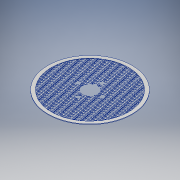
# Autodesk Inventor part: Ground_Antenna230mm_Reflector
Saved by Autodesk Inventor 2018 (Build 220112000, 112)
## iProperties
Created: 2018-09-26
Part Number: Ground_Antenna230mm_Reflector
Material: Aluminum 6061
Document SubType Name: Modeling
Designer: Bradley
Density: 2.7 g/cm^3
Appearance: Aluminum - Flat
Mass: 288.186 g
Surface Area: 2617.31 cm^2
Volume: 106.736 cm^3
Author: Bradley
Autodesk Inventor part; units mm, degrees
ref_plane "YZ Plane" through (0, 0, 0) normal (1, 0, 0) x (0, 1, 0)
ref_plane "XZ Plane" through (0, 0, 0) normal (0, 1, 0) x (-1, 0, 0)
ref_plane "XY Plane" through (0, 0, 0) normal (0, 0, 1) x (1, 0, 0)
sketch "Sketch1" plane through (0, 0, 0) normal (0, 0, 1) x (1, 0, 0)
  circle A0 centre (0, 0) radius 152.4
  circle A1 centre (0, 0) radius 139.7
  dimension "d0" = 304.8
  dimension "d1" = 279.4
  constraints: 2 centre point, 2 coincident
  measures "d0" diameter of A0
  measures "d1" diameter of A1
sketch "Sketch2" plane through (0, 0, 0) normal (0, 0, 1) x (1, 0, 0)
  line L0 (-152.4, 139.7) -> (152.4, 139.7)
  line L1 (152.4, 139.7) -> (152.4, 136.7)
  line L2 (152.4, 136.7) -> (-152.4, 136.7)
  line L3 (-152.4, 136.7) -> (-152.4, 139.7)
  circle A0 centre (0, 0) radius 139.7 projected
  line L4 (-152.4, 129.2) -> (152.4, 129.2)
  line L5 (152.4, 129.2) -> (152.4, 126.2)
  line L6 (152.4, 126.2) -> (-152.4, 126.2)
  line L7 (-152.4, 126.2) -> (-152.4, 129.2)
  line L8 (-152.4, 118.7) -> (152.4, 118.7)
  line L9 (152.4, 118.7) -> (152.4, 115.7)
  line L10 (152.4, 115.7) -> (-152.4, 115.7)
  line L11 (-152.4, 115.7) -> (-152.4, 118.7)
  line L12 (-152.4, 108.2) -> (152.4, 108.2)
  line L13 (152.4, 108.2) -> (152.4, 105.2)
  line L14 (152.4, 105.2) -> (-152.4, 105.2)
  line L15 (-152.4, 105.2) -> (-152.4, 108.2)
  line L16 (-152.4, 97.7) -> (152.4, 97.7)
  line L17 (152.4, 97.7) -> (152.4, 94.7)
  line L18 (152.4, 94.7) -> (-152.4, 94.7)
  line L19 (-152.4, 94.7) -> (-152.4, 97.7)
  line L20 (-152.4, 87.2) -> (152.4, 87.2)
  line L21 (152.4, 87.2) -> (152.4, 84.2)
  line L22 (152.4, 84.2) -> (-152.4, 84.2)
  line L23 (-152.4, 84.2) -> (-152.4, 87.2)
  line L24 (-152.4, 76.7) -> (152.4, 76.7)
  line L25 (152.4, 76.7) -> (152.4, 73.7)
  line L26 (152.4, 73.7) -> (-152.4, 73.7)
  line L27 (-152.4, 73.7) -> (-152.4, 76.7)
  line L28 (-152.4, 66.2) -> (152.4, 66.2)
  line L29 (152.4, 66.2) -> (152.4, 63.2)
  line L30 (152.4, 63.2) -> (-152.4, 63.2)
  line L31 (-152.4, 63.2) -> (-152.4, 66.2)
  line L32 (-152.4, 55.7) -> (152.4, 55.7)
  line L33 (152.4, 55.7) -> (152.4, 52.7)
  line L34 (152.4, 52.7) -> (-152.4, 52.7)
  line L35 (-152.4, 52.7) -> (-152.4, 55.7)
  line L36 (-152.4, 45.2) -> (152.4, 45.2)
  line L37 (152.4, 45.2) -> (152.4, 42.2)
  line L38 (152.4, 42.2) -> (-152.4, 42.2)
  line L39 (-152.4, 42.2) -> (-152.4, 45.2)
  point P0 (0, 139.7)
  point P1 (0, 129.2)
  point P2 (0, 118.7)
  point P3 (0, 108.2)
  point P4 (0, 97.7)
  point P5 (0, 87.2)
  point P6 (0, 76.7)
  point P7 (0, 66.2)
  point P8 (0, 55.7)
  point P9 (0, 45.2)
  dimension "d2" = 304.8
  dimension "d3" = 3
  dimension "d6" = 10.5
  constraints: 80 end point, 2 parallel, 1 collinear, 1 horizontal, 1 midpoint, 1 perpendicular, 1 tangent, 1 vertical, 1 vertical alignment, 80 other
  measures "d2" distance of L0.start L0.end
  measures "d3" distance of L0.end L1.end
  measures "d6" distance of L0.start L4.start
extrude "Extrusion1" add sketch "Sketch2" along normal mid plane 0.75 contours L0 A0 L2 L3 | L0 L1 L2 A0 | A0 L2 | L4 L5 L6 A0 | A0 L6 L4 | A0 L6 L7 L4 | L8 L9 L10 A0 | A0 L10 L8 | A0 L10 L11 L8 | L12 L13 L14 A0 | A0 L14 L12 | A0 L14 L15 L12 | L16 L17 L18 A0 | A0 L18 L16 | A0 L18 L19 L16 | L20 L21 L22 A0 | A0 L22 L20 | A0 L22 L23 L20 | L24 L25 L26 A0 | A0 L26 L24 | A0 L26 L27 L24 | L28 L29 L30 A0 | A0 L30 L28 | A0 L30 L31 L28 | L32 L33 L34 A0 | A0 L34 L32 | A0 L34 L35 L32 | L36 L37 L38 A0 | A0 L38 L36 | A0 L38 L39 L36
pattern_linear "Rectangular Pattern1" count 3 spacing 105 along (0, -1, 0) of "Extrusion1"
sketch "Sketch3" plane through (0, 0, 0) normal (0, 0, 1) x (1, 0, 0)
  line L0 (-201.8323, 44.7837) -> (62.1323, 197.1837)
  line L1 (62.1323, 197.1837) -> (63.6323, 194.5857)
  line L2 (63.6323, 194.5857) -> (-200.3323, 42.1857)
  line L3 (-200.3323, 42.1857) -> (-201.8323, 44.7837)
  line L4 (152.4, 139.7) -> (-152.4, 139.7) projected
  line L5 (152.4, 136.7) -> (152.4, 139.7) projected
  circle A0 centre (0, 0) radius 139.7 projected
  line L6 (0, 0) -> (-69.85, 120.9837)
  line L7 (-196.5823, 35.6905) -> (67.3823, 188.0905)
  line L8 (67.3823, 188.0905) -> (68.8823, 185.4924)
  line L9 (68.8823, 185.4924) -> (-195.0823, 33.0924)
  line L10 (-195.0823, 33.0924) -> (-196.5823, 35.6905)
  line L11 (-191.3323, 26.5972) -> (72.6323, 178.9972)
  line L12 (72.6323, 178.9972) -> (74.1323, 176.3991)
  line L13 (74.1323, 176.3991) -> (-189.8323, 23.9991)
  line L14 (-189.8323, 23.9991) -> (-191.3323, 26.5972)
  line L15 (-186.0823, 17.5039) -> (77.8823, 169.9039)
  line L16 (77.8823, 169.9039) -> (79.3823, 167.3059)
  line L17 (79.3823, 167.3059) -> (-184.5823, 14.9059)
  line L18 (-184.5823, 14.9059) -> (-186.0823, 17.5039)
  line L19 (-180.8323, 8.4107) -> (83.1323, 160.8107)
  line L20 (83.1323, 160.8107) -> (84.6323, 158.2126)
  line L21 (84.6323, 158.2126) -> (-179.3323, 5.8126)
  line L22 (-179.3323, 5.8126) -> (-180.8323, 8.4107)
  line L23 (-175.5823, -0.6826) -> (88.3823, 151.7174)
  line L24 (88.3823, 151.7174) -> (89.8823, 149.1193)
  line L25 (89.8823, 149.1193) -> (-174.0823, -3.2807)
  line L26 (-174.0823, -3.2807) -> (-175.5823, -0.6826)
  line L27 (-170.3323, -9.7759) -> (93.6323, 142.6241)
  line L28 (93.6323, 142.6241) -> (95.1323, 140.0261)
  line L29 (95.1323, 140.0261) -> (-168.8323, -12.3739)
  line L30 (-168.8323, -12.3739) -> (-170.3323, -9.7759)
  line L31 (-165.0823, -18.8691) -> (98.8823, 133.5309)
  line L32 (98.8823, 133.5309) -> (100.3823, 130.9328)
  line L33 (100.3823, 130.9328) -> (-163.5823, -21.4672)
  line L34 (-163.5823, -21.4672) -> (-165.0823, -18.8691)
  line L35 (-159.8323, -27.9624) -> (104.1323, 124.4376)
  line L36 (104.1323, 124.4376) -> (105.6323, 121.8395)
  line L37 (105.6323, 121.8395) -> (-158.3323, -30.5605)
  line L38 (-158.3323, -30.5605) -> (-159.8323, -27.9624)
  line L39 (-154.5823, -37.0557) -> (109.3823, 115.3443)
  line L40 (109.3823, 115.3443) -> (110.8823, 112.7463)
  line L41 (110.8823, 112.7463) -> (-153.0823, -39.6537)
  line L42 (-153.0823, -39.6537) -> (-154.5823, -37.0557)
  point P0 (-64.6, 111.8905)
  point P1 (-59.35, 102.7972)
  point P2 (-54.1, 93.7039)
  point P3 (-48.85, 84.6107)
  point P4 (-43.6, 75.5174)
  point P5 (-38.35, 66.4241)
  point P6 (-33.1, 57.3309)
  point P7 (-27.85, 48.2376)
  point P8 (-22.6, 39.1443)
  dimension "d23" = 30
  dimension "d26" = 10.5
  constraints: 82 end point, 2 equal length, 2 parallel, 1 collinear, 1 midpoint, 1 perpendicular, 84 other
  measures "d23" angle of L0 L4
  measures "d26" distance of L0.start L7.start
extrude "Extrusion4" add sketch "Sketch3" along normal mid plane 0.75 contours L0 A0 L2 L3 | L0 L4 L2 A0 | L6 L2 A0 | A0 L2 L6 | L0 L1 L2 L4 | L7 L4 L9 A0 | A0 L9 L6 L7 | L7 L6 L9 A0 | A0 L9 L10 L7 | L7 L8 L9 L4 | L11 L6 L13 A0 | A0 L13 L14 L11 | L11 A0 L13 L6 | L11 L12 L13 L4 | L4 L13 A0 L11 | L15 L6 L17 A0 | A0 L17 L18 L15 | L15 A0 L17 L6 | L15 L16 L17 L4 | L4 L17 A0 L15 | L19 L6 L21 A0 | A0 L21 L22 L19 | L19 A0 L21 L6 | L19 L20 L21 L4 | L4 L21 A0 L19 | L23 L6 L25 A0 | A0 L25 L26 L23 | L23 A0 L25 L6 | L23 L24 L25 L4 | L4 L25 A0 L23 | L27 L6 L29 A0 | A0 L29 L30 L27 | L27 A0 L29 L6 | L27 L28 L29 L4 | L4 L29 A0 L27 | L31 L6 L33 A0 | A0 L33 L34 L31 | L31 A0 L33 L6 | L31 L32 L33 A0 | L35 L6 L37 A0 | A0 L37 L38 L35 | L35 A0 L37 L6 | L35 L36 L37 A0 | L39 L6 L41 A0 | A0 L41 L42 L39 | L39 A0 L41 L6 | L39 L40 L41 A0
pattern_linear "Rectangular Pattern2" count 3 spacing 105 along (0.5, -0.866, 0) of "Extrusion4"
extrude "Extrusion2" cut sketch "Sketch1" along normal through all both and the other way through all contours A1 keep common part
extrude "Extrusion3" add sketch "Sketch1" along normal mid plane 2
sketch "Sketch4" plane through (0, 0, 0) normal (0, 0, 1) x (1, 0, 0)
  circle A0 centre (0, 0) radius 27.5
  circle A1 centre (-43.6562, 0) radius 7.9375
  circle A2 centre (0, -43.6562) radius 7.9375
  circle A3 centre (43.6562, 0) radius 7.9375
  circle A4 centre (0, 43.6562) radius 7.9375
  dimension "d36" = 55
  dimension "d41" = 360
  dimension "d43" = 87.3125
  dimension "d44" = 15.875
  constraints: 5 centre point, 1 coincident, 1 horizontal alignment, 9 other
  measures "d36" diameter of A0
  measures "d43" distance of A3.centre A1.centre
  measures "d44" diameter of A1
extrude "Extrusion5" cut sketch "Sketch4" along normal through all both and the other way through all
equation "\"d2\" = d0"
equation "\"d6\" = 3.5 * d3"
equation "\"d15\" = 10 * d6"
equation "\"d26\" = d6"
equation "\"d31\" = d11"
equation "\"d35\" = 10 * d6"
equation "\"d11\" = 0.75"
body "Solid1"
